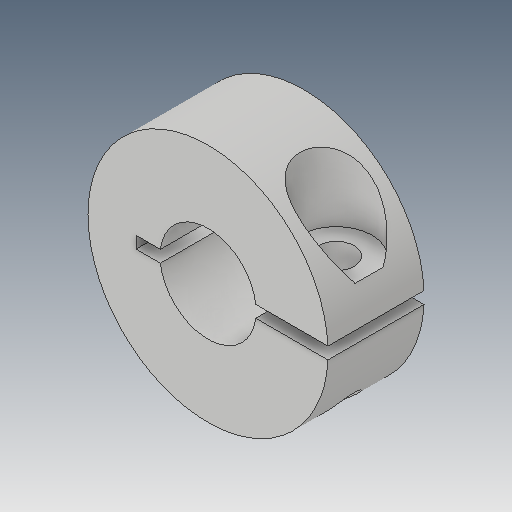
# Autodesk Inventor part: セットカラー
Saved by Autodesk Inventor 2020.3 (Build 243373000, 373)
## iProperties
Part Number: セットカラー
Material: 一般
Document SubType Name: Modeling
Designer: highs
Density: 1 g/cm^3
Appearance: 既定
Stock Number: 要調査
Author: highs
Autodesk Inventor part; units mm, degrees
ref_plane "YZ Plane" through (0, 0, 0) normal (1, 0, 0) x (0, 1, 0)
ref_plane "XY Plane" through (0, 0, 0) normal (0, 0, 1) x (1, 0, 0)
sketch "スケッチ1" plane through (0, 0, 0) normal (0, 0, 1) x (1, 0, 0)
  circle A0 centre (0, 0) radius 15
  circle A1 centre (0, 0) radius 6
  dimension "d0" = 30
  dimension "d1" = 12
  constraints: 2 centre point, 2 coincident
  measures "d0" diameter of A0
  measures "d1" diameter of A1
extrude "押し出し1" add sketch "スケッチ1" along normal blind 12
sketch "スケッチ2" plane through (0, 0, 0) normal (0, 1, 0) x (-1, 0, 0)
  line L0 (0, 0) -> (0, 12) construction
  line L1 (0, 6) -> (-10, 6) construction
  circle A0 centre (-10, 6) radius 2.25
  line L2 (15, 12) -> (-15, 12) construction
  line L3 (-15, 0) -> (15, 0) construction
  dimension "d4" = 4.5
  dimension "d5" = 10
  dimension "d6" = 6
  constraints: 4 end point, 1 centre point, 1 coincident, 1 horizontal, 1 midpoint, 1 vertical
  measures "d4" diameter of A0
  measures "d5" distance of L1.start L1.end
  measures "d6" distance between parallel lines of L3 L1
extrude "押し出し2" cut sketch "スケッチ2" along normal through all both and the other way through all
sketch "スケッチ3" plane through (0, 0, 12) normal (0, 0, 1) x (1, 0, 0)
  line L0 (0, 0) -> (-15.0903, 0) construction
  line L1 (-9, 0.75) -> (21, 0.75)
  line L2 (21, 0.75) -> (21, -0.75)
  line L3 (21, -0.75) -> (-9, -0.75)
  line L4 (-9, -0.75) -> (-9, 0.75)
  line L5 (-9, 0.75) -> (21, -0.75) construction
  line L6 (21, 0.75) -> (-9, -0.75) construction
  point P0 (6, 0)
  dimension "d9" = 9
  dimension "d10" = 1.5
  dimension "d11" = 30
  constraints: 14 end point, 2 horizontal, 2 midpoint, 2 parallel, 1 perpendicular, 1 point on line
  measures "d9" distance from line of L4 L0.start
  measures "d10" distance of L3.end L1.start
  measures "d11" distance of L2.end L3.end
extrude "押し出し3" cut sketch "スケッチ3" against normal through all
ref_plane "作業平面1" through (0, 5, 0) normal (0, 1, 0) x (-1, 0, 0)
sketch "スケッチ4" plane through (0, 5, 0) normal (0, 1, 0) x (-1, 0, 0)
  circle A0 centre (-9.9953, 6) radius 4.5
  line L0 (0, 0) -> (0.0094, 12) construction
  line L1 (15, 12) -> (-14.9812, 12) construction
  line L2 (0.0047, 6) -> (-9.9953, 6) construction
  dimension "d15" = 9
  dimension "d16" = 10
  constraints: 4 end point, 2 midpoint, 1 centre point, 1 horizontal
  measures "d15" diameter of A0
  measures "d16" distance of L2.start L2.end
extrude "押し出し4" cut sketch "スケッチ4" along normal through all
